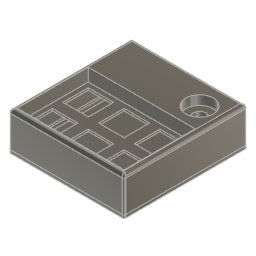
3by2 rotary v7 (Autodesk Fusion 360 design; units mm, degrees)
Autodesk Fusion 360 part; units mm, degrees
note: some values were not read from the file. Set by a fixed rule: which sketch regions a step uses.
sketch "Sketch1" plane through (0, 0, 0) normal (0, 0, 1) x (1, 0, 0)
  line L0 (1, 0) -> (61.8, 0)
  line L1 (62.8, 1) -> (62.8, 66.0607)
  line L2 (61.8, 67.0607) -> (1, 67.0607)
  line L3 (0, 66.0607) -> (0, 1)
  line L4 (5, 5) -> (18.8, 5)
  line L5 (18.8, 5) -> (18.8, 18.8)
  line L6 (18.8, 18.8) -> (5, 18.8)
  line L7 (5, 18.8) -> (5, 5)
  line L8 (38.3, 18.8) -> (24.5, 18.8)
  line L9 (24.5, 18.8) -> (24.5, 5)
  line L10 (38.3, 5) -> (38.3, 18.8)
  line L11 (24.5, 5) -> (38.3, 5)
  line L12 (57.8, 18.8) -> (44, 18.8)
  line L13 (44, 18.8) -> (44, 5)
  line L14 (57.8, 5) -> (57.8, 18.8)
  line L15 (44, 5) -> (57.8, 5)
  line L16 (18.8, 38.3) -> (5, 38.3)
  line L17 (5, 38.3) -> (5, 24.5)
  line L18 (18.8, 24.5) -> (18.8, 38.3)
  line L19 (5, 24.5) -> (18.8, 24.5)
  line L20 (38.3, 38.3) -> (24.5, 38.3)
  line L21 (24.5, 38.3) -> (24.5, 24.5)
  line L22 (38.3, 24.5) -> (38.3, 38.3)
  line L23 (24.5, 24.5) -> (38.3, 24.5)
  line L24 (57.8, 38.3) -> (44, 38.3)
  line L25 (44, 38.3) -> (44, 24.5)
  line L26 (57.8, 24.5) -> (57.8, 38.3)
  line L27 (44, 24.5) -> (57.8, 24.5)
  line L28 (2, 61.5603) -> (35.81, 61.5603)
  line L29 (35.81, 61.5603) -> (35.81, 43.3603)
  line L30 (35.81, 43.3603) -> (2, 43.3603)
  line L31 (35.3999, 45.3501) -> (6, 45.3501)
  line L32 (6, 59.5501) -> (35.3999, 59.5501)
  line L33 (37.3999, 63.6019) -> (37.3999, 41.3501)
  line L34 (37.3999, 41.3501) -> (31.9039, 41.3501)
  line L35 (31.9039, 43.3603) -> (31.9039, 41.3501)
  line L36 (31.8901, 61.5603) -> (31.8901, 63.6019)
  line L37 (33.4999, 47.2503) -> (7.9001, 47.2503)
  line L38 (7.9001, 57.65) -> (33.4999, 57.65)
  line L39 (33.4999, 57.65) -> (35.81, 57.65)
  line L40 (7.9001, 57.65) -> (2, 57.6034)
  line L41 (7.9001, 47.2503) -> (2, 47.3114)
  line L42 (33.4999, 47.2503) -> (35.81, 47.2503)
  line L43 (6, 59.5501) -> (2, 59.5501)
  line L44 (35.3999, 59.5501) -> (35.81, 59.5501)
  line L45 (6, 45.3501) -> (2, 45.3501)
  line L46 (35.3999, 45.3501) -> (35.81, 45.3501)
  arc A0 (0, 1) -> (1, 0) centre (1, 1) ccw
  arc A1 (61.8, 0) -> (62.8, 1) centre (61.8, 1) ccw
  arc A2 (62.8, 66.0607) -> (61.8, 67.0607) centre (61.8, 66.0607) ccw
  arc A3 (1, 67.0607) -> (0, 66.0607) centre (1, 66.0607) ccw
  line L47 (2, 63.6019) -> (-0.7188, 63.6019)
  line L48 (31.8901, 63.6019) -> (37.3999, 63.6019)
  line L49 (2.3, 41) -> (60.5, 41)
  line L50 (60.5, 41) -> (60.5, 2.3)
  line L51 (60.5, 2.3) -> (2.3, 2.3)
  line L52 (2.3, 2.3) -> (2.3, 41)
  line L53 (2, 2) -> (60.8, 2)
  line L54 (60.8, 2) -> (60.8, 65.0607)
  line L55 (60.8, 65.0607) -> (2, 65.0607)
  line L56 (2, 65.0607) -> (2, 2)
  circle A4 centre (38.4086, 53.1111) radius 2
  arc A5 (35.81, 50.2751) -> (35.81, 55.947) centre (38.4086, 53.1111) ccw
  circle A6 centre (50.9, 52.9756) radius 3.5
  line L57 (58.4, 60.4756) -> (43.4, 60.4756)
  line L58 (43.4, 60.4756) -> (43.4, 45.4756)
  line L59 (43.4, 45.4756) -> (58.4, 45.4756)
  line L60 (58.4, 45.4756) -> (58.4, 60.4756)
  line L61 (58.4, 60.4756) -> (43.4, 45.4756) construction
  line L62 (43.4, 60.4756) -> (58.4, 45.4756) construction
  point P0 (50.9, 38.3)
  point P1 (50.9, 52.9756)
  dimension "d1" = 13.8
  dimension "d2" = 13.8
  dimension "d6" = 19.5
  dimension "d7" = 19.5
  dimension "d9" = 5
  dimension "d10" = 5
  dimension "d11" = 5
  dimension "d13" = -2
  dimension "d90" = 33.81
  dimension "d91" = 18.2
  dimension "d108" = 1
  dimension "d122" = 67.0607
  dimension "d130" = 2.7
  dimension "d131" = 2.7
  dimension "d132" = 2.7
  dimension "d133" = 2.7
  dimension "d191" = 4
  dimension "d197" = 7
  dimension "d214" = 15
  dimension "d215" = 15
  constraint horizontal L0
  constraint vertical L1
  constraint horizontal L2
  constraint vertical L3
  constraint horizontal L4
  constraint vertical L5
  constraint horizontal L6
  constraint vertical L7
  constraint horizontal L28
  constraint vertical L29
  constraint horizontal L30
  constraint coincident L30 L35.start
  constraint perpendicular L34 L35
  constraint coincident L28 L36.start
  constraint coincident L36.end L47
  constraint perpendicular L36 L47
  constraint coincident L29 L39.end
  constraint perpendicular L29 L39
  constraint coincident L29 L42.end
  constraint perpendicular L29 L42
  constraint horizontal L43
  constraint coincident L29 L44.end
  constraint perpendicular L29 L44
  constraint horizontal L45
  constraint coincident L45.end L56
  constraint coincident L29 L46.end
  constraint perpendicular L29 L46
  constraint tangent L0 A0
  constraint tangent L3 A0
  constraint tangent L0 A1
  constraint tangent L1 A1
  constraint equal A0 A1
  constraint tangent L1 A2
  constraint tangent L2 A2
  constraint equal A0 A2
  constraint tangent L2 A3
  constraint tangent L3 A3
  constraint equal A0 A3
  constraint coincident origin L0
  constraint coincident origin L3
  constraint parallel L30 L37
  constraint parallel L28 L38
  constraint parallel L30 L31
  constraint parallel L28 L32
  constraint parallel L28 L47
  constraint parallel L29 L33
  constraint parallel L30 L34
  constraint coincident L41.end L56
  constraint coincident L40.end L56
  constraint coincident L28.start L56
  constraint coincident L30.end L56
  constraint coincident L43.end L56
  constraint collinear L47 L48
  constraint horizontal L49
  constraint vertical L50
  constraint horizontal L51
  constraint vertical L52
  constraint concentric A4 A5
  constraint coincident L29 A5.end
  constraint coincident L29 A5.start
  constraint midpoint L24 P0
  constraint vertical P1 P0
  constraint horizontal L57
  constraint perpendicular L57 L58
  constraint parallel L57 L59
  constraint parallel L58 L60
  constraint coincident L61 P1
  constraint coincident L62 P1
  constraint coincident P1 A6.centre
  measures "d1" distance of L4.start L4.end
  measures "d2" distance of L4.start L6.end
  measures "d9" distance of L0 L4
  measures "d10" distance of L3 L7
  measures "d11" distance of L1 L14
  measures "d90" distance of L28.start L28.end
  measures "d91" distance of L28.start L30.end
  measures "d108" radius of A0
  measures "d122" distance of L0 L2
  measures "d130" distance of L16 L49
  measures "d131" distance of L17 L52
  measures "d132" distance of L26 L50
  measures "d133" distance of L11 L51
  measures "d191" diameter of A4
  measures "d197" diameter of A6
  measures "d214" distance of L58.end L59.end
  measures "d215" distance of L57.end L58.end
extrude "Extrude1" add sketch "Sketch1" along normal blind 1.2 contours L0 L1 L2 L3 A0 A1 A2 A3 | L28 L30 L33 L34 L35 L36 L48 L53 L54 L55 L56 A5 | L28 L29 L32 L43 L44 L56 | L28 L29 L33 L36 L48 A5 | L29 L32 L38 L39 L40 L43 L44 L56 | L29 L37 L38 L39 L40 L41 L42 L56 | L29 L31 L37 L41 L42 L45 L46 L56 | L33 A4 A5 | L29 L33 A4 A5 | L29 L30 L31 L45 L46 L56 | L33 A4 | L33 A4 | L29 L30 L33 L34 L35 A5 | L49 L50 L51 L52 | A6 | L57 L58 L59 L60 makes body 1
extrude "Extrude6" add sketch "Sketch1" against normal blind 11 contours L0 L1 L2 L3 A0 A1 A2 A3 bodies 1
extrude "Extrude20" add sketch "Sketch1" against normal blind 3 contours L28 L29 L33 L36 L48 A5 | L29 L33 A4 A5 | L33 A4 | L29 L30 L33 L34 L35 A5 picked at (37.0769, 53.0122) bodies 1
extrude "Extrude21" add sketch "Sketch1" against normal blind 1.5 contours L29 L32 L38 L39 L40 L43 L44 L56 | L29 L31 L37 L41 L42 L45 L46 L56 bodies 1
sketch "Sketch9" plane through (2, 0, 0) normal (1, 0, 0) x (0, 1, 0)
  line L0 (2, -11) -> (65.0607, -11)
  line L1 (50.6154, -6) -> (54.6154, -6)
  arc A0 (54.6154, -6) -> (54.6154, -2) centre (54.6154, -4) ccw
  line L2 (54.6154, -2) -> (50.6154, -2)
  arc A1 (50.6154, -2) -> (50.6154, -6) centre (50.6154, -4) ccw
  line L3 (48.6154, -4) -> (56.6154, -4) construction
  line L4 (66.0607, 0) -> (1, 0)
  line L5 (45.3501, 0) -> (2, 0)
  line L6 (47.3114, 0) -> (47.3114, -1.5)
  line L7 (47.3114, -1.5) -> (45.3501, -1.5)
  line L8 (45.3501, -1.5) -> (45.3501, 0)
  line L9 (65.0607, 0) -> (59.5501, 0)
  line L10 (59.5501, 0) -> (59.5501, -1.5)
  line L11 (59.5501, -1.5) -> (57.6034, -1.5)
  line L12 (57.6034, -1.5) -> (57.6034, 0)
  line L13 (57.6034, 0) -> (47.3114, 0)
  line L14 (2, 0) -> (2, -11)
  line L15 (65.0607, -11) -> (65.0607, 0)
  dimension "d100" = 4
  dimension "d104" = 2
  constraint tangent L1 A0
  constraint tangent A0 L2
  constraint parallel L1 L2
  constraint tangent L2 A1
  constraint tangent L1 A1
  constraint midpoint A1 L3.start
  constraint midpoint A0 L3.end
  measures "d100" diameter of A0
  measures "d104" distance of L2 L4
extrude "Extrude22" cut sketch "Sketch9" against normal blind 8 contours L1 A0 L2 A1 bodies 1
sketch "Sketch10" plane through (0, 0, -11) normal (0, 0, -1) x (1, 0, 0)
  line L0 (2, -2) -> (60.8, -2)
  line L1 (60.8, -2) -> (60.8, -65.0607)
  line L2 (60.8, -65.0607) -> (2, -65.0607)
  line L3 (2, -65.0607) -> (2, -2)
  arc A0 (0, -66.0607) -> (1, -67.0607) centre (1, -66.0607) ccw
  line L4 (1, -67.0607) -> (61.8, -67.0607)
  arc A1 (61.8, -67.0607) -> (62.8, -66.0607) centre (61.8, -66.0607) ccw
  line L5 (62.8, -66.0607) -> (62.8, -1)
  arc A2 (62.8, -1) -> (61.8, 0) centre (61.8, -1) ccw
  line L6 (61.8, 0) -> (1, 0)
  arc A3 (1, 0) -> (0, -1) centre (1, -1) ccw
  line L7 (0, -1) -> (0, -66.0607)
  arc A4 (60.75, -4) -> (58.8, -2.05) centre (58.8, -4) ccw
  line L8 (4, -2.05) -> (58.8, -2.05)
  arc A5 (4, -2.05) -> (2.05, -4) centre (4, -4) ccw
  line L9 (2.05, -63.0607) -> (2.05, -4)
  arc A6 (2.05, -63.0607) -> (4, -65.0107) centre (4, -63.0607) ccw
  line L10 (58.8, -65.0107) -> (4, -65.0107)
  arc A7 (58.8, -65.0107) -> (60.75, -63.0607) centre (58.8, -63.0607) ccw
  line L11 (60.75, -4) -> (60.75, -63.0607)
  arc A8 (59.6, -4) -> (58.8, -3.2) centre (58.8, -4) ccw
  line L12 (4, -3.2) -> (58.8, -3.2)
  arc A9 (4, -3.2) -> (3.2, -4) centre (4, -4) ccw
  line L13 (3.2, -63.0607) -> (3.2, -4)
  arc A10 (3.2, -63.0607) -> (4, -63.8607) centre (4, -63.0607) ccw
  line L14 (58.8, -63.8607) -> (4, -63.8607)
  arc A11 (58.8, -63.8607) -> (59.6, -63.0607) centre (58.8, -63.0607) ccw
  line L15 (59.6, -4) -> (59.6, -63.0607)
  line L16 (33.3999, -49.0564) -> (37.3999, -49.0564)
  line L17 (37.3999, -49.0564) -> (37.3999, -56.0564)
  line L18 (37.3999, -56.0564) -> (33.3999, -56.0564)
  line L19 (33.3999, -56.0564) -> (33.3999, -49.0564)
  line L20 (35.81, -61.5603) -> (35.81, -43.3603)
  line L21 (37.3999, -63.6019) -> (37.3999, -41.3501)
  line L22 (33.4999, -57.65) -> (35.81, -57.65)
  line L23 (2, -61.5603) -> (35.81, -61.5603)
  dimension "d117" = 7
  dimension "d118" = 4
  dimension "d119" = 5.5039
  constraint horizontal L16
  constraint vertical L17
  constraint horizontal L18
  constraint vertical L19
  constraint coincident L17.end L21
  constraint parallel L0 L8
  constraint parallel L3 L9
  constraint parallel L2 L10
  constraint parallel L1 L11
  constraint tangent A6 L10
  constraint tangent A4 L11
  constraint tangent A7 L11
  constraint tangent A4 L8
  constraint tangent L8 A5
  constraint tangent A5 L9
  constraint tangent L10 A7
  constraint tangent L9 A6
  constraint parallel L0 L12
  constraint parallel L3 L13
  constraint parallel L2 L14
  constraint parallel L1 L15
  constraint tangent A10 L14
  constraint tangent A8 L15
  constraint tangent A8 L12
  constraint tangent L12 A9
  constraint tangent A11 L15
  constraint tangent A9 L13
  constraint tangent L13 A10
  constraint tangent L14 A11
  measures "d117" distance of L16 L18
  measures "d118" distance of L17 L19
  measures "d119" distance of L18 L23
extrude "Extrude23" add sketch "Sketch10" along normal blind 1.6 separate body contours L0 L1 L2 L3 | A0 L4 A1 L5 A2 L6 A3 L7 | A4 L8 A5 L9 A6 L10 A7 L11 | A8 L12 A9 L13 A10 L14 A11 L15 | L16 L18 L19 L20 | L16 L17 L18 L20 L21 makes body 2
extrude "Extrude24" add sketch "Sketch10" against normal blind 2 contours A4 L8 A5 L9 A6 L10 A7 L11 bodies 2
fillet "Fillet8" radius 1 6 edges at (31.9039, 41.3501, -1.5) (31.9039, 43.3603, -1.5) (37.3999, 41.3501, -1.5) (37.3999, 63.6019, -1.5) (31.8901, 63.6019, -1.5) (31.8901, 61.5603, -1.5) on bodies 1
extrude "Extrude26" add sketch "Sketch1" along normal blind 7 from surface at 1.2 contours L0 L1 L2 L3 A0 A1 A2 A3 | L28 L30 L33 L34 L35 L36 L48 L53 L54 L55 L56 A5 | L28 L29 L32 L43 L44 L56 | L28 L29 L33 L36 L48 A5 | L29 L32 L38 L39 L40 L43 L44 L56 | L29 L37 L38 L39 L40 L41 L42 L56 | L29 L31 L37 L41 L42 L45 L46 L56 | L33 A4 A5 | L29 L33 A4 A5 | L29 L30 L31 L45 L46 L56 | L33 A4 | L33 A4 | L29 L30 L33 L34 L35 A5 | A6 | L57 L58 L59 L60 bodies 1
sketch "Sketch12" plane through (0, 0, 0) normal (-1, 0, 0) x (0, -1, 0)
  line L0 (-50.6154, -6) -> (-54.6154, -6)
  arc A0 (-54.6154, -2) -> (-54.6154, -6) centre (-54.6154, -4) ccw
  line L1 (-54.6154, -2) -> (-50.6154, -2)
  arc A1 (-50.6154, -6) -> (-50.6154, -2) centre (-50.6154, -4) ccw
  line L2 (-1, -11) -> (-1, 8.2)
  line L3 (-1, 8.2) -> (-66.0607, 8.2)
  line L4 (-66.0607, 8.2) -> (-66.0607, -11)
  line L5 (-66.0607, -11) -> (-1, -11)
  line L6 (-67.0607, 8.2) -> (-67.0607, -11)
  line L7 (-66.0607, 8.2) -> (-1, 8.2)
  line L8 (-41, 8.2) -> (-2.3, 8.2)
  line L9 (-2.3, 8.2) -> (-41, 8.2)
  line L10 (-66.0607, 8.2) -> (-67.0607, 8.2)
  line L11 (-66.0607, 8.2) -> (-1, 8.2)
  line L12 (0, 8.2) -> (-1, 8.2)
  line L13 (0, 8.2) -> (-1, 8.2)
  line L14 (-1, 8.2) -> (-66.0607, 8.2)
  line L15 (-66.0607, 8.2) -> (-67.0607, 8.2)
  line L16 (-41.5863, 8.2) -> (-67.0607, 3.2)
  line L17 (-67.0607, 8.2) -> (-41.5863, 8.2)
  point P0 (-41, 8.2)
  dimension "d144" = 5
  constraint coincident L11 L16.start
  constraint coincident L6 L16.end
  constraint coincident L6.start L10.end
  measures "d144" distance of L16.end L17
extrude "Extrude30" add sketch "Sketch1" against normal up to surface (3 mm away) contours L33 A4 A5 bodies 1
extrude "Extrude31" cut sketch "Sketch1" along normal blind -4.5 and the other way blind -5 contours L33 A4 | L33 A4 bodies 1
extrude "Extrude32" cut sketch "Sketch1" along normal up to surface (8.2 mm away) contours A6 bodies 1
sketch "Sketch14" plane through (0, 0, 8.2) normal (0, 0, 1) x (-1, 0, 0)
  circle A0 centre (-50.9, -52.9756) radius 3.5
  line L0 (-60.5, -41) -> (-60.5, -2.3)
  line L1 (-60.5, -2.3) -> (-2.3, -2.3)
  line L2 (-2.3, -2.3) -> (-2.3, -41)
  line L3 (-2.3, -41) -> (-60.5, -41)
  line L4 (-61.8, -67.0607) -> (-1, -67.0607)
  arc A1 (-1, -67.0607) -> (0, -66.0607) centre (-1, -66.0607) ccw
  line L5 (0, -66.0607) -> (0, -1)
  arc A2 (0, -1) -> (-1, 0) centre (-1, -1) ccw
  line L6 (-1, 0) -> (-61.8, 0)
  arc A3 (-61.8, 0) -> (-62.8, -1) centre (-61.8, -1) ccw
  line L7 (-62.8, -1) -> (-62.8, -66.0607)
  arc A4 (-62.8, -66.0607) -> (-61.8, -67.0607) centre (-61.8, -66.0607) ccw
  circle A5 centre (-50.9, -52.9756) radius 7.5
  point P0 (-50.9, -52.9756)
  dimension "d200" = 15
  constraint concentric A0 A5
  measures "d200" diameter of A5
extrude "Extrude33" cut sketch "Sketch14" against normal blind 5 contours A5 bodies 1
fillet "Fillet17" radius 2 8 edges at (31.4, 67.0607, 8.2) (0.2929, 66.7678, 8.2) (0, 33.5303, 8.2) (0.2929, 0.2929, 8.2) (31.4, 0, 8.2) (62.5071, 0.2929, 8.2) (62.8, 33.5303, 8.2) (62.5071, 66.7678, 8.2) on bodies 1
fillet "Fillet18" radius 1.5 4 edges at (0, 52.6154, -6) (0, 56.6154, -4) (0, 52.6154, -2) (0, 48.6154, -4) on bodies 1
sketch "Sketch15" plane through (62.8, 0, 0) normal (1, 0, 0) x (0, 1, 0)
  line L0 (66.0607, 6.2) -> (1, 6.2)
  line L1 (1, 6.2) -> (1, -11)
  line L2 (1, -11) -> (66.0607, -11)
  line L3 (66.0607, -11) -> (66.0607, 6.2)
  line L4 (2, 0) -> (2, -11)
  line L5 (65.0607, 0) -> (65.0607, -11)
  circle A0 centre (2, -9) radius 1
  circle A1 centre (65.0607, -9) radius 0.8
  circle A2 centre (65.0607, -9) radius 0.5
  circle A3 centre (2, -9) radius 0.5
  line L6 (1.697, -9.3977) -> (2.05, -9.9766)
  line L7 (2.05, -11) -> (2.05, -9)
  line L8 (2.05, -9) -> (2.05, -11)
  line L9 (2.05, -9.3977) -> (2.05, -9.9766)
  line L10 (1.697, -9.3977) -> (2.05, -9.3977)
  dimension "d209" = 2
  dimension "d210" = 1.6
  dimension "d223" = 1
  dimension "d224" = 1
  dimension "d229" = 2
  constraint coincident L4 A0.centre
  constraint coincident L5 A1.centre
  constraint horizontal A0.centre A1.centre
  constraint concentric A1 A2
  constraint concentric A0 A3
  constraint coincident A3 L6.start
  constraint coincident L6.end L7
  constraint coincident L7 L9.start
  constraint parallel L7 L9
  constraint perpendicular L7 L10
  measures "d209" diameter of A0
  measures "d210" diameter of A1
  measures "d223" diameter of A2
  measures "d224" diameter of A3
  measures "d229" distance of L4.end A0.centre
extrude "Extrude34" cut sketch "Sketch15" against normal up to surface (58.8 mm away) from surface at -2 contours L4 A0 A3 L6 | L4 A3 L10 | L4 A3 L6 | L4 A3 L10 | L5 A1 A2 | L5 A2 picked at (65.4886, -9.5518) picked at (65.3083, -8.874) bodies 1
extrude "Extrude35" add sketch "Sketch15" against normal up to surface (54.2 mm away) from surface at -4.3 contours L4 A3 L7 L8 L9 L10 | L4 A3 L10 | L4 A3 L6 | L4 A3 L6 L7 L8 L9 | L4 A3 L7 L8 L9 L10 | L4 A3 L10 | L5 A2 | L5 A2 bodies 2
fillet "Fillet19" radius 1.25 2 edges at (31.4, 2.5, -9) (31.4, 64.5607, -9) on bodies 2
equation "d1 = keyWidth"
equation "d2 = keyWidth"
equation "keyWidth = 13.8 mm"
equation "d6 = keySpacing"
equation "d7 = keySpacing"
equation "keySpacing = keyWidth + 5.7 mm"
equation "d10 = d9"
equation "d11 = d10"
equation "d90 = PromicroLength + 0.2 mm"
equation "PromicroLength = 33.61 mm"
equation "d131 = d130"
equation "d132 = d130"
equation "d133 = d130"
equation "bottomPlateTolerance = 0.05 mm"
equation "d210 = d223 + 0.6 mm"
named bodies: "3by2 case rotary", "3by2 tpop backplate"
